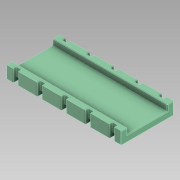
# Autodesk Inventor part: TrussCC_box
Saved by Autodesk Inventor 2021 (Build 250183000, 183)
## iProperties
Created: 2021-02-11
Part Number: TrussCC_box
Material: 一般
Document SubType Name: Modeling
Designer: kumagai
Density: 1 g/cm^3
Appearance: 滑らか - 濃い海緑
Author: kumagai
Autodesk Inventor part; units mm, degrees
ref_plane "YZ Plane" through (0, 0, 0) normal (1, 0, 0) x (0, 1, 0)
ref_plane "XZ Plane" through (0, 0, 0) normal (0, 1, 0) x (-1, 0, 0)
ref_plane "XY Plane" through (0, 0, 0) normal (0, 0, 1) x (1, 0, 0)
sketch "スケッチ2" plane through (0, 0, 0) normal (1, 0, 0) x (0, 1, 0)
  line L0 (-8.4, 0) -> (8.4, 0) projected
  line L1 (0, 35) -> (0, -35) projected
  line L2 (6, 19.1) -> (0, 19.1)
  line L3 (0, 19.1) -> (0, -19.1)
  line L4 (0, -19.1) -> (6, -19.1)
  line L5 (6, -19.1) -> (6, -25)
  line L6 (6, -25) -> (-6, -25)
  line L7 (-6, -25) -> (-6, 25)
  line L8 (-6, 25) -> (6, 25)
  line L9 (6, 25) -> (6, 19.1)
  point P0 (0, 0)
  dimension "d0" = 50
  dimension "d1" = 6
  dimension "d2" = 38.2
  dimension "d3" = 6
  constraints: 16 end point, 4 perpendicular, 3 horizontal, 3 point on line, 2 other
  measures "d0" distance between parallel lines of L6 L8
  measures "d1" distance between parallel lines of L3 L9
  measures "d2" distance between parallel lines of L4 L2
  measures "d3" distance between parallel lines of L7 L1
extrude "押し出し1" add sketch "スケッチ2" along normal mid plane 110
sketch "スケッチ3" plane through (0, 0, 0) normal (1, 0, 0) x (0, 1, 0)
  line L0 (7, 22) -> (-2, 22)
  line L1 (-2, 22) -> (-2, -22)
  line L2 (-2, -22) -> (7, -22)
  line L3 (7, -22) -> (7, -26)
  line L4 (7, -26) -> (-7, -26)
  line L5 (-7, -26) -> (-7, 26)
  line L6 (-7, 26) -> (7, 26)
  line L7 (7, 26) -> (7, 22)
  line L8 (0, 36.4) -> (0, -36.4) projected
  line L9 (-9.8, 0) -> (9.8, 0) projected
  line L10 (6, 25) -> (6, 19.1) projected
  line L11 (-6, 25) -> (6, 25) projected
  line L12 (-6, -25) -> (-6, 25) projected
  point P0 (0, 0)
  dimension "d6" = 2
  dimension "d7" = 22
  dimension "d8" = 1
  dimension "d9" = 1
  dimension "d10" = 1
  constraints: 16 end point, 7 perpendicular, 1 collinear, 1 horizontal, 2 other
  measures "d6" distance between parallel lines of L1 L8
  measures "d7" distance between parallel lines of L2 L9
  measures "d8" distance between parallel lines of L7 L10
  measures "d9" distance between parallel lines of L6 L11
  measures "d10" distance between parallel lines of L12 L5
extrude "押し出し2" cut sketch "スケッチ3" along normal mid plane 4.8 contours L0 L10 L11 L8 L6 L7 | L0 L8 L11 L10 | L0 L1 L9 L12 L11 L8 | L8 L11 L12 L9 L5 L6 | L1 L2 L8 L4 L5 L9 | L2 L3 L4 L8
pattern_linear "矩形状パターン1" count 5 spacing 23 along (1, 0, 0) of "押し出し2" first direction both ways yes
chamfer "面取り1" distance 0.4 angle 45 24 edges at (43.6, -6, 0) (34.5, -6, 25) (25.4, -6, 0) (34.5, -6, -25) (51.7, -6, 25) (55, -6, 0) (48.4, -6, 0) (51.7, -6, -25) (11.5, -6, 25) (20.6, -6, 0) (2.4, -6, 0) (11.5, -6, -25) (-2.4, -6, 0) (-11.5, -6, 25) (-20.6, -6, 0) (-11.5, -6, -25) (-25.4, -6, 0) (-34.5, -6, 25) (-43.6, -6, 0) (-34.5, -6, -25) (-51.7, -6, 25) (-48.4, -6, 0) (-55, -6, 0) (-51.7, -6, -25)
chamfer "面取り2" distance 0.6 angle 45 16 edges at (55, 0.2, 25) (55, 3, 19.1) (55, 0, 0) (55, 3, -19.1) (55, 0.2, -25) (-55, 0.2, 25) (-55, 0.2, -25) (-55, 3, -19.1) (-55, 0, 0) (-55, 3, 19.1) (-55, 6, 22.05) (55, 6, 22.05) (0, 6, 19.1) (55, 6, -22.05) (0, 6, -19.1) (-55, 6, -22.05)
